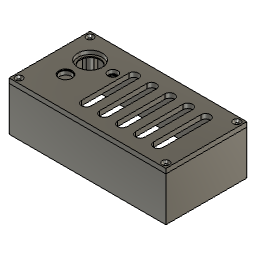
LED Panel Top (Autodesk Fusion 360 design; units mm, degrees)
Autodesk Fusion 360 part; units mm, degrees
sketch "Sketch5" plane through (0, 0, 0) normal (0, 0, 1) x (-1, 0, 0)
  line L0 (-80.25, -40.25) -> (-80.25, 40.25)
  line L1 (-80.25, 40.25) -> (80.25, 40.25)
  line L2 (80.25, 40.25) -> (80.25, -40.25)
  line L3 (80.25, -40.25) -> (-80.25, -40.25)
  line L4 (82.71, -42.71) -> (82.71, 42.71)
  line L5 (82.71, 42.71) -> (-82.71, 42.71)
  line L6 (-82.71, 42.71) -> (-82.71, -42.71)
  line L7 (-82.71, -42.71) -> (82.71, -42.71)
  line L8 (-80.25, 40.25) -> (80.25, 40.25)
  line L9 (80.25, 40.25) -> (80.25, -40.25)
  line L10 (80.25, -40.25) -> (-80.25, -40.25)
  line L11 (-80.25, -40.25) -> (-80.25, 40.25)
  line L12 (-80.25, 40.25) -> (80.25, -40.25) construction
  line L13 (80.25, 40.25) -> (-80.25, -40.25) construction
  line L14 (-82.71, 42.71) -> (82.71, 42.71)
  line L15 (82.71, 42.71) -> (82.71, -42.71)
  line L16 (82.71, -42.71) -> (-82.71, -42.71)
  line L17 (-82.71, -42.71) -> (-82.71, 42.71)
  line L18 (-82.71, 42.71) -> (82.71, -42.71) construction
  line L19 (82.71, 42.71) -> (-82.71, -42.71) construction
  line L20 (80.25, -40.25) -> (72.25, -40.25)
  line L21 (72.25, -40.25) -> (72.25, -32.25)
  line L22 (72.25, -32.25) -> (80.25, -32.25)
  line L23 (80.25, -32.25) -> (80.25, -40.25)
  line L24 (80.25, -40.25) -> (72.25, -32.25) construction
  line L25 (72.25, -40.25) -> (80.25, -32.25) construction
  circle A0 centre (77.48, -37.48) radius 2.2
  line L26 (66.5, -36) -> (58.5, -36)
  line L27 (58.5, -40.25) -> (58.5, -28)
  line L28 (58.5, -28) -> (66.5, -28)
  line L29 (66.5, -28) -> (66.5, -40.25)
  line L30 (66.5, -36) -> (58.5, -28) construction
  line L31 (58.5, -36) -> (66.5, -28) construction
  circle A1 centre (62.5, -32) radius 1.75
  line L32 (0, 0) -> (0, -11.7816) construction
  line L33 (0, 0) -> (-11.8343, 0) construction
  line L34 (-72.25, -40.25) -> (-80.25, -32.25) construction
  line L35 (-80.25, -40.25) -> (-72.25, -40.25)
  circle A2 centre (-77.48, -37.48) radius 2.2
  circle A3 centre (-62.5, -32) radius 1.75
  line L36 (-58.5, -28) -> (-66.5, -28)
  line L37 (-66.5, -36) -> (-58.5, -36)
  line L38 (-80.25, -32.25) -> (-80.25, -40.25)
  line L39 (-72.25, -40.25) -> (-72.25, -32.25)
  line L40 (-66.5, -36) -> (-58.5, -28) construction
  line L41 (-58.5, -40.25) -> (-58.5, -28)
  line L42 (-72.25, -32.25) -> (-80.25, -32.25)
  line L43 (-80.25, -40.25) -> (-72.25, -32.25) construction
  line L44 (-58.5, -36) -> (-66.5, -28) construction
  line L45 (-66.5, -23.75) -> (-66.5, -40.25)
  line L46 (72.25, 40.25) -> (80.25, 32.25) construction
  line L47 (58.5, 40.25) -> (58.5, 28)
  line L48 (66.5, 28) -> (66.5, 40.25)
  line L49 (80.25, 32.25) -> (80.25, 40.25)
  circle A4 centre (77.48, 37.48) radius 2.2
  line L50 (58.5, 28) -> (66.5, 28)
  line L51 (72.25, 40.25) -> (72.25, 32.25)
  line L52 (72.25, 32.25) -> (80.25, 32.25)
  line L53 (58.5, 36) -> (66.5, 28) construction
  line L54 (66.5, 36) -> (58.5, 36)
  line L55 (80.25, 40.25) -> (72.25, 32.25) construction
  circle A5 centre (62.5, 32) radius 1.75
  line L56 (80.25, 40.25) -> (72.25, 40.25)
  line L57 (66.5, 36) -> (58.5, 28) construction
  line L58 (-58.5, 36) -> (-66.5, 28) construction
  line L59 (-80.25, 32.25) -> (-80.25, 40.25)
  line L60 (-66.5, 23.75) -> (-66.5, 40.25)
  line L61 (-80.25, 40.25) -> (-72.25, 40.25)
  circle A6 centre (-77.48, 37.48) radius 2.2
  line L62 (-72.25, 40.25) -> (-80.25, 32.25) construction
  line L63 (-72.25, 32.25) -> (-80.25, 32.25)
  line L64 (-58.5, 28) -> (-66.5, 28)
  line L65 (-66.5, 36) -> (-58.5, 28) construction
  line L66 (-66.5, 36) -> (-58.5, 36)
  line L67 (-80.25, 40.25) -> (-72.25, 32.25) construction
  line L68 (-58.5, 40.25) -> (-58.5, 28)
  line L69 (-72.25, 40.25) -> (-72.25, 32.25)
  circle A7 centre (-62.5, 32) radius 1.75
  line L70 (82.71, -42.71) -> (72.25, -32.25) construction
  line L71 (72.25, -42.71) -> (82.71, -32.25) construction
  circle A8 centre (-50.25, 28.75) radius 2
  circle A9 centre (-50.25, -28.75) radius 2
  line L72 (-50.25, 28.75) -> (-50.25, 26.8205) construction
  line L73 (-50.25, -28.75) -> (-50.25, -5.4886) construction
  line L74 (-50.25, 28.75) -> (-50.25, -28.75) construction
  line L75 (-66.5, 23.75) -> (-45.25, 23.75)
  line L76 (-45.25, 23.75) -> (-45.25, 33.75)
  line L77 (-45.25, 33.75) -> (-55.25, 33.75)
  line L78 (-55.25, 33.75) -> (-55.25, 23.75)
  line L79 (-55.25, 23.75) -> (-45.25, 33.75) construction
  line L80 (-45.25, 23.75) -> (-55.25, 33.75) construction
  line L81 (-55.25, -33.75) -> (-45.25, -33.75)
  line L82 (-45.25, -33.75) -> (-45.25, -23.75)
  line L83 (-45.25, -23.75) -> (-66.5, -23.75)
  line L84 (-55.25, -23.75) -> (-55.25, -33.75)
  line L85 (-55.25, -33.75) -> (-45.25, -23.75) construction
  line L86 (-45.25, -33.75) -> (-55.25, -23.75) construction
  line L87 (-45.25, -33.75) -> (-45.25, -40.25)
  line L88 (-55.25, -33.75) -> (-55.25, -40.25)
  line L89 (-45.25, 33.75) -> (-45.25, 40.25)
  line L90 (-55.25, 33.75) -> (-55.25, 40.25)
  point P0 (-82.71, -42.71)
  point P1 (-80.25, -40.25)
  point P2 (-80.25, -40.25)
  point P3 (-82.71, -42.71)
  point P4 (82.71, 42.71)
  point P5 (80.25, 40.25)
  point P6 (80.25, 40.25)
  point P7 (-80.25, 40.25)
  point P8 (-80.25, 40.25)
  point P9 (-80.25, 40.25)
  point P10 (-80.25, 40.25)
  point P11 (-50.25, 28.75)
  point P12 (-50.25, -28.75)
  dimension "d75" = 160.5
  dimension "d76" = 80.5
  dimension "d77" = 165.42
  dimension "d78" = 85.42
  dimension "d79" = 8
  dimension "d80" = 8
  dimension "d81" = 4.4
  dimension "d82" = 8
  dimension "d83" = 8
  dimension "d84" = 3.5
  dimension "d85" = 8.25
  dimension "d86" = 17.75
  dimension "d124" = 4
  dimension "d125" = 4
  dimension "d126" = 57.5
  dimension "d127" = 28.75
  dimension "d128" = 30
  dimension "d129" = 10
  dimension "d130" = 10
  dimension "d131" = 10
  dimension "d132" = 10
  constraint horizontal L8
  constraint perpendicular L8 L9
  constraint parallel L8 L10
  constraint parallel L9 L11
  constraint coincident L12 L32.start
  constraint coincident L13 L32.start
  constraint coincident L32.start L33.start
  constraint horizontal L14
  constraint perpendicular L14 L15
  constraint parallel L14 L16
  constraint parallel L15 L17
  constraint coincident L18 L32.start
  constraint coincident L19 L32.start
  constraint horizontal L20
  constraint vertical L21
  constraint horizontal L22
  constraint vertical L23
  constraint coincident L2.end L3.start
  constraint horizontal L26
  constraint vertical L27
  constraint horizontal L28
  constraint vertical L29
  constraint midpoint L30 A1.centre
  constraint coincident L3 L29.end
  constraint coincident L26.start L29
  constraint coincident L3 L27.start
  constraint coincident L26.end L27
  constraint vertical L32
  constraint horizontal L33
  constraint symmetric L2.end L32 P2
  constraint symmetric L4.start L32 P3
  constraint symmetric L20.end L32 L34.start
  constraint symmetric L21.end L32 L39.end
  constraint symmetric L22.end L32 L34.end
  constraint symmetric A0 L32 A2
  constraint symmetric L26.start L32 L37.start
  constraint symmetric L26.end L32 L37.end
  constraint symmetric L27.end L32 L36.start
  constraint symmetric L28.end L32 L36.end
  constraint symmetric A1 L32 A3
  constraint symmetric L29.end L32 L45.end
  constraint symmetric L27.start L32 L41.start
  constraint symmetric P2 L33 P10
  constraint symmetric L2.end L33 P6
  constraint symmetric L4.start L33 P4
  constraint symmetric L20.end L33 L46.start
  constraint symmetric L21.end L33 L51.end
  constraint symmetric L22.end L33 L46.end
  constraint symmetric A0 L33 A4
  constraint symmetric L26.start L33 L54.start
  constraint symmetric L26.end L33 L53.start
  constraint symmetric L27.end L33 L47.end
  constraint symmetric L28.end L33 L48.start
  constraint symmetric A1 L33 A5
  constraint symmetric L29.end L33 L48.end
  constraint symmetric L27.start L33 L47.start
  constraint symmetric L33 L36.end L58.end
  constraint symmetric L33 L37.start L65.start
  constraint symmetric L33 L34.end L59.start
  constraint symmetric L33 L39.end L63.start
  constraint symmetric L33 P2 P10
  constraint symmetric L33 L34.start L61.end
  constraint symmetric L33 L41.start L68.start
  constraint symmetric L33 L45.end L60.end
  constraint symmetric L33 L37.end L58.start
  constraint symmetric L33 L36.start L64.start
  constraint symmetric L33 A2 A6
  constraint symmetric L33 A3 A7
  constraint coincident L24 A0.centre
  constraint coincident L16 L71.start
  constraint coincident L15 L71.end
  constraint perpendicular L70 L71
  constraint midpoint A0.centre L71
  constraint coincident P11 A8.centre
  constraint vertical L72
  constraint coincident P12 A9.centre
  constraint vertical L73
  constraint collinear L72 L73
  constraint horizontal L75
  constraint perpendicular L75 L76
  constraint parallel L75 L77
  constraint parallel L76 L78
  constraint coincident L79 P11
  constraint coincident L80 P11
  constraint horizontal L81
  constraint perpendicular L81 L82
  constraint parallel L81 L83
  constraint parallel L82 L84
  constraint coincident L85 P12
  constraint coincident L86 P12
  constraint coincident L10 L87.end
  constraint perpendicular L10 L87
  constraint coincident L10 L88.end
  constraint perpendicular L10 L88
  constraint coincident L1 L89.end
  constraint perpendicular L1 L89
  constraint coincident L1 L90.end
  constraint perpendicular L1 L90
  constraint coincident L78.end L75
  constraint coincident L58.end L60
  constraint coincident L84.start L83
  constraint coincident L36.end L45
  measures "d75" distance of L2.end P2
  measures "d76" distance of P6 L2.end
  measures "d77" distance of L4.start P3
  measures "d78" distance of P4 L4.start
  measures "d79" distance of L2.end L20.end
  measures "d80" distance of L2.end L22.end
  measures "d81" diameter of A0
  measures "d82" distance of L26.start L26.end
  measures "d83" distance of L26.start L28.end
  measures "d84" diameter of A1
  measures "d85" distance of L10 A1.centre
  measures "d86" distance of L9 A1.centre
  measures "d124" diameter of A8
  measures "d125" diameter of A9
  measures "d126" distance of P11 P12
  measures "d127" distance of L33 P12
  measures "d128" distance of L0 L74
  measures "d129" distance of L76.end L77.end
  measures "d130" distance of L75.end L76.end
  measures "d131" distance of L82.end L84.start
  measures "d132" distance of L81.end L82.end
extrude "Extrude4" add sketch "Sketch5" along normal blind 30 contours L0 L3 L10 L11 L35 L38 L39 L42 | L0 L1 L8 L11 L59 L61 L63 L69 | L2 L3 L9 L10 L20 L21 L22 L23 | L1 L2 L8 L9 L49 L51 L52 L56 | L4 L5 L6 L7 L14 L15 L16 L17 | A0 | A2 | A4 | A6 makes body 1
extrude "Extrude13" add sketch "Sketch5" against normal blind 16.5 contours L4 L5 L6 L7 L14 L15 L16 L17 bodies 1
chamfer "Chamfer2" distance 2.46 angle 45 4 edges at (0, -40.25, -16.5) (-80.25, 0, -16.5) (0, 40.25, -16.5) (80.25, 0, -16.5) on bodies 1
extrude "Extrude7" cut sketch "Sketch5" against normal blind 8 from surface at 30 contours A0 | A2 | A4 | A6 bodies 1
extrude "Extrude5" add sketch "Sketch5" along normal blind 5 contours L3 L10 L37 L41 L45 | L3 L10 L36 L41 L45 L83 L84 L88 | L36 L37 L41 L45 | L3 L10 L81 L87 L88 | L1 L8 L60 L66 L68 | L81 L82 L83 L84 | L1 L8 L60 L64 L68 L75 L78 L90 | L60 L64 L66 L68 | L3 L10 L26 L27 L29 | L1 L8 L77 L89 L90 | L26 L27 L28 L29 | L75 L76 L77 L78 | L1 L8 L47 L48 L54 | L47 L48 L50 L54 bodies 1
fillet "Fillet6" radius 4 8 edges at (-58.5, -28, 2.5) (-66.5, -28, 2.5) (-66.5, 28, 2.5) (-58.5, 28, 2.5) (45.25, 23.75, 2.5) (66.5, 23.75, 2.5) (45.25, -23.75, 2.5) (66.5, -23.75, 2.5) on bodies 1
fillet "Fillet8" radius 4 4 edges at (-72.25, -32.25, 15) (-72.25, 32.25, 15) (72.25, 32.25, 15) (72.25, -32.25, 15) on bodies 1
sketch "Sketch6" plane through (0, 0, 30) normal (0, 0, 1) x (-1, 0, 0)
  circle A0 centre (77.48, -37.48) radius 2.2
  circle A1 centre (-77.48, 37.48) radius 2.2
  circle A2 centre (77.48, 37.48) radius 2.2
  circle A3 centre (-77.48, -37.48) radius 2.2
  line L0 (72.25, 40.25) -> (72.25, 36.25)
  line L1 (76.25, 32.25) -> (80.25, 32.25)
  line L2 (80.25, 32.25) -> (80.25, -32.25)
  line L3 (80.25, -32.25) -> (76.25, -32.25)
  line L4 (72.25, -36.25) -> (72.25, -40.25)
  line L5 (72.25, -40.25) -> (-72.25, -40.25)
  line L6 (-72.25, -40.25) -> (-72.25, -36.25)
  line L7 (-76.25, -32.25) -> (-80.25, -32.25)
  line L8 (-80.25, -32.25) -> (-80.25, 32.25)
  line L9 (-80.25, 32.25) -> (-76.25, 32.25)
  line L10 (-72.25, 36.25) -> (-72.25, 40.25)
  line L11 (-82.71, -42.71) -> (82.71, -42.71)
  line L12 (82.71, -42.71) -> (82.71, 42.71)
  line L13 (82.71, 42.71) -> (-82.71, 42.71)
  line L14 (-82.71, 42.71) -> (-82.71, -42.71)
  line L15 (-82.71, 42.71) -> (82.71, 42.71)
  line L16 (82.71, 42.71) -> (82.71, -42.71)
  line L17 (82.71, -42.71) -> (-82.71, -42.71)
  line L18 (-82.71, -42.71) -> (-82.71, 42.71)
  line L19 (-82.71, 42.71) -> (82.71, -42.71) construction
  line L20 (82.71, 42.71) -> (-82.71, -42.71) construction
  circle A4 centre (77.48, -37.48) radius 1.75
  circle A5 centre (77.48, 37.48) radius 1.75
  circle A6 centre (-77.48, -37.48) radius 1.75
  circle A7 centre (-77.48, 37.48) radius 1.75
  circle A8 centre (32.25, -16.25) radius 5.075
  circle A9 centre (32.25, -16.25) radius 4
  arc A10 (-76.25, 32.25) -> (-72.25, 36.25) centre (-76.25, 36.25) ccw
  line L21 (-72.25, 40.25) -> (72.25, 40.25)
  arc A11 (72.25, 36.25) -> (76.25, 32.25) centre (76.25, 36.25) ccw
  arc A12 (76.25, -32.25) -> (72.25, -36.25) centre (76.25, -36.25) ccw
  arc A13 (-72.25, -36.25) -> (-76.25, -32.25) centre (-76.25, -36.25) ccw
  circle A14 centre (56.25, -16.25) radius 13
  circle A15 centre (56.25, -16.25) radius 10.5
  circle A16 centre (56.25, 9.675) radius 6.25
  circle A17 centre (56.25, 9.675) radius 7
  line L22 (-14, 25) -> (-14, -25)
  line L23 (-24, -25) -> (-24, 25)
  line L24 (-24, 0) -> (-14, 0) construction
  line L25 (-19, 0) -> (-19, 8.6843) construction
  line L26 (-5, 0) -> (5, 0) construction
  line L27 (5, 25) -> (5, -25)
  line L28 (0, 0) -> (0, 6.9936) construction
  line L29 (-5, -25) -> (-5, 25)
  line L30 (0, -2.5) -> (0, -20)
  line L31 (24, -25) -> (24, 25)
  line L32 (14, 25) -> (14, -25)
  arc A18 (-19, 30) -> (-24, 25) centre (-19, 25) ccw
  arc A19 (-14, 25) -> (-19, 30) centre (-19, 25) ccw
  arc A20 (-24, -25) -> (-19, -30) centre (-19, -25) ccw
  arc A21 (-19, -30) -> (-14, -25) centre (-19, -25) ccw
  arc A22 (0, 30) -> (-5, 25) centre (0, 25) ccw
  arc A23 (5, 25) -> (0, 30) centre (0, 25) ccw
  arc A24 (-5, -25) -> (0, -30) centre (0, -25) ccw
  arc A25 (0, -30) -> (5, -25) centre (0, -25) ccw
  arc A26 (19, 30) -> (14, 25) centre (19, 25) ccw
  arc A27 (24, 25) -> (19, 30) centre (19, 25) ccw
  arc A28 (14, -25) -> (19, -30) centre (19, -25) ccw
  arc A29 (19, -30) -> (24, -25) centre (19, -25) ccw
  line L33 (-14, 25) -> (-14, -25)
  line L34 (-24, 0) -> (-14, 0) construction
  arc A30 (-24, -25) -> (-19, -30) centre (-19, -25) ccw
  line L35 (-24, -25) -> (-24, 25)
  arc A31 (-19, 30) -> (-24, 25) centre (-19, 25) ccw
  arc A32 (-19, -30) -> (-14, -25) centre (-19, -25) ccw
  arc A33 (-14, 25) -> (-19, 30) centre (-19, 25) ccw
  line L36 (-19, 0) -> (-19, 8.6843) construction
  arc A34 (-57, 30) -> (-62, 25) centre (-57, 25) ccw
  line L37 (-43, 0) -> (-33, 0) construction
  line L38 (-57, 0) -> (-57, 8.6843) construction
  line L39 (-52, 25) -> (-52, -25)
  arc A35 (-38, 30) -> (-43, 25) centre (-38, 25) ccw
  arc A36 (-38, -30) -> (-33, -25) centre (-38, -25) ccw
  arc A37 (-33, 25) -> (-38, 30) centre (-38, 25) ccw
  arc A38 (-62, -25) -> (-57, -30) centre (-57, -25) ccw
  line L40 (-33, 25) -> (-33, -25)
  arc A39 (-57, -30) -> (-52, -25) centre (-57, -25) ccw
  line L41 (-38, 0) -> (-38, 8.6843) construction
  line L42 (-62, -25) -> (-62, 25)
  line L43 (-62, 0) -> (-52, 0) construction
  line L44 (-43, -25) -> (-43, 25)
  arc A40 (-52, 25) -> (-57, 30) centre (-57, 25) ccw
  arc A41 (-43, -25) -> (-38, -30) centre (-38, -25) ccw
  point P0 (-24, 30)
  point P1 (-14, 30)
  point P2 (-24, -30)
  point P3 (-5, -30)
  point P4 (5, 30)
  point P5 (-5, 30)
  point P6 (-24, -30)
  point P7 (-14, 30)
  point P8 (-24, 30)
  point P9 (-62, -30)
  point P10 (-52, 30)
  point P11 (-43, -30)
  point P12 (-62, 30)
  point P13 (-33, 30)
  point P14 (-43, 30)
  dimension "d102" = 165.42
  dimension "d103" = 85.42
  dimension "d104" = 3.5
  dimension "d105" = 3.5
  dimension "d106" = 3.5
  dimension "d107" = 3.5
  dimension "d110" = 10.15
  dimension "d111" = 8
  dimension "d143" = 24
  dimension "d144" = 48
  dimension "d145" = 26
  dimension "d146" = 21
  dimension "d147" = 24
  dimension "d148" = 24
  dimension "d149" = 12.5
  dimension "d150" = 14
  dimension "d151" = 24
  dimension "d152" = 49.925
  dimension "d154" = 10
  dimension "d155" = 60
  dimension "d158" = 42.71
  dimension "d160" = 10
  dimension "d161" = 60
  dimension "d162" = 14
  dimension "d163" = 5
  dimension "d164" = 5
  dimension "d165" = 5
  dimension "d166" = 5
  dimension "d167" = 5
  dimension "d168" = 5
  dimension "d169" = 5
  dimension "d170" = 5
  dimension "d171" = 5
  dimension "d172" = 10
  dimension "d173" = 60
  dimension "d174" = 5
  dimension "d175" = 5
  dimension "d176" = 10
  dimension "d177" = 60
  dimension "d178" = 5
  dimension "d179" = 5
  dimension "d180" = 10
  dimension "d181" = 60
  dimension "d182" = 5
  dimension "d183" = 5
  dimension "d184" = 19
  dimension "d185" = 19
  constraint horizontal L15
  constraint perpendicular L15 L16
  constraint parallel L15 L17
  constraint parallel L16 L18
  constraint coincident L19 L28.start
  constraint coincident L20 L28.start
  constraint coincident L28.start origin
  constraint concentric A0 A4
  constraint concentric A2 A5
  constraint concentric A3 A6
  constraint concentric A1 A7
  constraint concentric A8 A9
  constraint concentric A14 A15
  constraint concentric A16 A17
  constraint vertical L22
  constraint vertical L23
  constraint midpoint L24 L25.start
  constraint perpendicular L24 L25
  constraint vertical L27
  constraint vertical L29
  constraint midpoint L28.start L26
  constraint perpendicular L26 L28
  constraint coincident L23 L24.start
  constraint coincident P8 L23
  constraint tangent L23 A18
  constraint coincident L22 L24.end
  constraint coincident P7 L22
  constraint tangent L22 A19
  constraint equal A18 A19
  constraint coincident A18.start A19.end
  constraint coincident P6 L23
  constraint tangent L23 A20
  constraint equal A18 A20
  constraint tangent L22 A21
  constraint coincident A20.end A21.start
  constraint coincident L26.start L29
  constraint coincident P5 L29
  constraint tangent L29 A22
  constraint coincident L26.end L27
  constraint coincident P4 L27
  constraint tangent L27 A23
  constraint coincident A22.start A23.end
  constraint coincident P3 L29
  constraint tangent L29 A24
  constraint tangent L27 A25
  constraint coincident A24.end A25.start
  constraint tangent L32 A26
  constraint tangent L31 A27
  constraint coincident A26.start A27.end
  constraint tangent L32 A28
  constraint tangent L31 A29
  constraint equal A28 A29
  constraint coincident A28.end A29.start
  constraint vertical L33
  constraint vertical L35
  constraint midpoint L25.start L34
  constraint perpendicular L34 L36
  constraint coincident L24.start L35
  constraint coincident P8 L35
  constraint tangent L35 A31
  constraint coincident L24.end L33
  constraint coincident P7 L33
  constraint tangent L33 A33
  constraint equal A31 A33
  constraint coincident P6 L35
  constraint tangent A30 L35
  constraint equal A30 A31
  constraint tangent L33 A32
  constraint vertical L40
  constraint vertical L44
  constraint midpoint L41.start L37
  constraint perpendicular L37 L41
  constraint coincident L37.start L44
  constraint coincident P14 L44
  constraint tangent A35 L44
  constraint coincident L37.end L40
  constraint coincident P13 L40
  constraint tangent A37 L40
  constraint equal A35 A37
  constraint coincident A35.start A37.end
  constraint coincident P11 L44
  constraint tangent L44 A41
  constraint equal A35 A41
  constraint tangent A36 L40
  constraint coincident A36.start A41.end
  constraint vertical L39
  constraint vertical L42
  constraint midpoint L38.start L43
  constraint perpendicular L38 L43
  constraint coincident L43.start L42
  constraint coincident P12 L42
  constraint tangent A34 L42
  constraint coincident L43.end L39
  constraint coincident P10 L39
  constraint tangent L39 A40
  constraint equal A34 A40
  constraint coincident A34.start A40.end
  constraint coincident P9 L42
  constraint tangent A38 L42
  constraint equal A34 A38
  constraint tangent L39 A39
  constraint coincident A38.end A39.start
  measures "d102" distance of L11.end L11.start
  measures "d103" distance of L12.end L11.end
  measures "d104" diameter of A4
  measures "d105" diameter of A5
  measures "d106" diameter of A6
  measures "d107" diameter of A7
  measures "d110" diameter of A8
  measures "d111" diameter of A9
  measures "d143" distance of L5 A8.centre
  measures "d144" distance of L2 A8.centre
  measures "d145" diameter of A14
  measures "d146" diameter of A15
  measures "d147" distance of L5 A14.centre
  measures "d148" distance of L2 A14.centre
  measures "d149" diameter of A16
  measures "d150" diameter of A17
  measures "d151" distance of L2 A16.centre
  measures "d152" distance of L5 A16.centre
  measures "d154" distance of P8 P7
  measures "d155" distance of P8 P6
  measures "d158" distance of L15 L24
  measures "d160" distance of P4 P5
  measures "d161" distance of P3 P5
  measures "d162" distance of L22 L30
  measures "d163" radius of A18
  measures "d164" radius of A21
  measures "d165" radius of A22
  measures "d166" radius of A23
  measures "d167" radius of A24
  measures "d168" radius of A25
  measures "d169" radius of A26
  measures "d170" radius of A27
  measures "d171" radius of A28
  measures "d172" distance of P7 P8
  measures "d173" distance of P6 P8
  measures "d174" radius of A31
  measures "d175" radius of A32
  measures "d176" distance of P13 P14
  measures "d177" distance of P11 P14
  measures "d178" radius of A35
  measures "d179" radius of A36
  measures "d180" distance of P10 P12
  measures "d181" distance of P9 P12
  measures "d182" radius of A34
  measures "d183" radius of A39
  measures "d184" distance of L25.start L41.start
  measures "d185" distance of L41.start L38.start
extrude "Extrude10" add sketch "Sketch6" along normal blind 5 separate body contours A0 | A1 | A2 | A3 | L0 L1 L2 L3 L4 L5 L6 L7 L8 L9 L10 A10 L21 A11 A12 A13 | L11 L12 L13 L14 L15 L16 L17 L18 | A8 | A14 | A17 makes body 2
extrude "Extrude11" cut sketch "Sketch6" against normal blind 4 from surface at 5 contours A8 | A14 | A15 bodies 2
extrude "Extrude15" cut sketch "Sketch6" against normal blind 1 from surface at 5 contours A17 bodies 2
chamfer "Chamfer3" distance 2 angle 45 4 edges at (79.1116, -38.1128, 35) (79.1116, 36.8472, 35) (-75.8484, -38.1128, 35) (-75.8484, 36.8472, 35) on bodies 2
equation "DisplayWidth = 160.5 mm"
equation "DisplayHeight = 80.5 mm"
equation "WallThickness = 2.46 mm"
equation "ScreenCoverThickness = 0.8 mm"
equation "P1WallHeight = 15 mm"
equation "P2Height = 30 mm"
equation "d46 = P2Height"
equation "d75 = DisplayWidth"
equation "d76 = DisplayHeight"
equation "d77 = DisplayWidth + 2 * WallThickness"
equation "d78 = DisplayHeight + 2 * WallThickness"
equation "d102 = DisplayWidth + 2 * WallThickness"
equation "d103 = DisplayHeight + 2 * WallThickness"
equation "d127 = ( 57.5 / 2 ) * 1 mm"
equation "d152 = 48 mm + 1.925 mm"
equation "d158 = ( 85.42 / 2 ) * 1 mm"
named bodies: "LED Panel Middle", "LED Panel Back"
